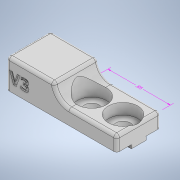
# Autodesk Inventor part: Mount Female V3
Saved by Autodesk Inventor 2020 (Build 240168000, 168)
## iProperties
Created: 2020-01-27
Part Number: Mount Female V3
Material: Generic
Document SubType Name: Modeling
Designer: maple
Density: 1 g/cm^3
Appearance: Default
Author: maple
Autodesk Inventor part; units mm, degrees
ref_plane "YZ Plane" through (0, 0, 0) normal (1, 0, 0) x (0, 1, 0)
ref_plane "XZ Plane" through (0, 0, 0) normal (0, 1, 0) x (-1, 0, 0)
ref_plane "XY Plane" through (0, 0, 0) normal (0, 0, 1) x (1, 0, 0)
sketch "Sketch1" plane through (0, 0, 0) normal (0, 1, 0) x (-1, 0, 0)
  line L0 (0, 0) -> (-38.1, 0)
  line L1 (-38.1, 0) -> (-38.1, -15.24)
  line L2 (-38.1, -15.24) -> (0, -15.24)
  line L3 (0, -15.24) -> (0, 0)
  dimension "d0" = 38.1
  dimension "d1" = 15.24
  constraints: 8 end point, 2 parallel, 1 horizontal, 1 perpendicular
  measures "d0" distance of L2.end L1.end
  measures "d1" distance of L1.end L0.end
extrude "Extrusion1" add sketch "Sketch1" along normal blind 5.08
sketch "Sketch2" plane through (0, 5.08, 0) normal (0, 1, 0) x (1, 0, 0)
  line L0 (0, 0) -> (16.51, 0)
  line L1 (16.51, 0) -> (16.51, 15.24)
  line L2 (16.51, 15.24) -> (0, 15.24)
  line L3 (0, 15.24) -> (0, 0)
  dimension "d4" = 16.51
  dimension "d5" = 15.24
  constraints: 8 end point, 2 parallel, 1 horizontal, 1 perpendicular
  measures "d4" distance of L2.end L1.end
  measures "d5" distance of L1.end L0.end
extrude "Extrusion2" add sketch "Sketch2" along normal blind 5.08
sketch "Sketch3" plane through (0, 0, -15.24) normal (-1, 0, 0) x (0, 0, 1)
  line L0 (0, 10.16) -> (15.24, 10.16) projected
  line L1 (7.62, 10.16) -> (7.62, 8.89)
  line L2 (7.62, 8.89) -> (2.54, 8.89)
  line L3 (2.54, 8.89) -> (2.54, 3.81)
  line L4 (2.54, 3.81) -> (12.7, 3.81)
  line L5 (12.7, 3.81) -> (12.7, 8.89)
  line L6 (12.7, 8.89) -> (7.62, 8.89)
  point P0 (15.24, 0)
  dimension "d8" = 1.27
  dimension "d9" = 5.08
  dimension "d10" = 5.08
  dimension "d11" = 10.16
  dimension "d12" = 90
  dimension "d13" = 5.08
  constraints: 12 end point, 2 perpendicular, 1 horizontal, 1 midpoint, 1 point on line, 1 vertical
  measures "d8" distance of L1.start L1.end
  measures "d9" distance of L1.end L2.end
  measures "d10" distance of L2.end L3.end
  measures "d11" distance of L3.end L4.end
  measures "d12" angle of L4 L3
  measures "d13" distance of L4.end L5.end
extrude "Extrusion3" cut sketch "Sketch3" against normal blind 15.24
sketch "Sketch4" plane through (0, 5.08, 0) normal (0, 1, 0) x (1, 0, 0)
  line L0 (38.1, 0) -> (38.1, 15.24) projected
  line L1 (38.1, 7.62) -> (32.7025, 7.62)
  line L2 (32.7025, 7.62) -> (27.305, 7.62)
  line L3 (27.305, 7.62) -> (21.8948, 7.62)
  point P0 (0, 0)
  dimension "d19" = 5.3975
  dimension "d20" = 5.3975
  dimension "d21" = 180
  dimension "d22" = 5.4102
  dimension "d23" = 180
  constraints: 6 end point, 2 collinear, 1 horizontal, 1 midpoint
  measures "d19" distance of L1.start L1.end
  measures "d20" distance of L1.end L2.end
  measures "d21" angle of L2 L1
  measures "d22" distance of L2.end L3.end
  measures "d23" angle of L3 L2
sketch "Sketch5" plane through (0, 0, 0) normal (0, -1, 0) x (1, 0, 0)
  line L0 (0, -15.24) -> (0, 0) projected
  line L1 (0, -7.62) -> (0, -10.16)
  line L2 (0, -10.16) -> (0, -5.08)
  line L3 (0, -5.08) -> (38.1, -5.08)
  line L4 (38.1, -5.08) -> (38.1, -10.16)
  line L5 (38.1, -10.16) -> (0, -10.16)
  line L6 (0, -10.16) -> (0, -5.08)
  dimension "d31" = 2.54
  dimension "d32" = 5.08
  dimension "d33" = 38.1
  dimension "d34" = 5.08
  constraints: 12 end point, 2 parallel, 2 point on line, 1 horizontal, 1 midpoint, 1 perpendicular
  measures "d31" distance of L1.start L1.end
  measures "d32" distance of L1.end L2.end
  measures "d33" distance of L4.end L5.end
  measures "d34" distance of L3.end L4.end
extrude "Extrusion4" add sketch "Sketch5" along normal blind 1.27
hole "Hole2" at (32.7025, 5.08, -7.62) at (21.8948, 5.08, -7.62) direction (0, -1, 0) diameter 5.08 end through all counterbore diameter 10.16 counterbore depth 3.81
fillet "Fillet1" radius 5.08 1 edges at (16.51, 5.08, -7.62)
fillet "Fillet2" radius 1.016 13 edges at (8.255, 10.16, 0) (8.255, 10.16, -15.24) (0, 5.08, -15.24) (0, 10.16, -7.62) (0, 5.08, 0) (16.51, 10.16, -7.62) (17.9979, 6.5679, 0) (29.845, 5.08, 0) (17.9979, 6.5679, -15.24) (29.845, 5.08, -15.24) (38.1, 5.08, -7.62) (38.1, 2.54, 0) (38.1, 2.54, -15.24)
fillet "Fillet3" radius 0.508 4 edges at (0, 3.81, -7.62) (0, 6.35, -2.54) (0, 6.35, -12.7) (0, 8.89, -7.62)
sketch "Sketch6" plane through (1.016, 0, 0) normal (0, 0, 1) x (1, 0, 0)
  line L0 (0.1598, 7.1739) -> (9.3236, 7.1739) construction
  line L1 (9.3236, 7.1739) -> (9.3236, 1.8798) construction
  line L2 (9.3236, 1.8798) -> (0.1598, 1.8798) construction
  line L3 (0.1598, 1.8798) -> (0.1598, 7.1739) construction
  line L4 (3.7352, 6.4319) -> (2.4261, 2.6219)
  line L5 (2.4261, 2.6219) -> (1.4288, 2.6219)
  line L6 (1.4288, 2.6219) -> (0.1197, 6.4319)
  line L7 (0.1197, 6.4319) -> (1.1108, 6.4319)
  line L8 (1.1108, 6.4319) -> (1.9413, 3.8476)
  line L9 (1.9413, 3.8476) -> (2.7688, 6.4319)
  line L10 (2.7688, 6.4319) -> (3.7352, 6.4319)
  spline S0 degree 2 poles (6.7856, 3.7766) (6.7856, 3.4956) (6.5788, 3.0356) (6.3781, 2.8751) knots 0 0 0 1 2 2 2
  spline S1 degree 2 poles (6.3781, 2.8751) (6.1774, 2.7145) (5.6309, 2.5416) (5.2388, 2.5416) knots 0 0 0 1 2 2 2
  spline S2 degree 2 poles (5.2388, 2.5416) (4.7942, 2.5416) (4.1582, 2.6898) (3.9575, 2.7824) knots 0 0 0 1 2 2 2
  line L11 (3.9575, 2.7824) -> (3.9575, 3.6099)
  line L12 (3.9575, 3.6099) -> (4.0501, 3.6099)
  spline S3 degree 2 poles (4.0501, 3.6099) (4.26, 3.4771) (4.8251, 3.2795) (5.0597, 3.2795) knots 0 0 0 1 2 2 2
  spline S4 degree 2 poles (5.0597, 3.2795) (5.1986, 3.2795) (5.5228, 3.3289) (5.634, 3.4092) knots 0 0 0 1 2 2 2
  spline S5 degree 2 poles (5.634, 3.4092) (5.7204, 3.474) (5.8254, 3.6624) (5.8254, 3.8322) knots 0 0 0 1 2 2 2
  spline S6 degree 2 poles (5.8254, 3.8322) (5.8254, 4.002) (5.6772, 4.1842) (5.5537, 4.2274) knots 0 0 0 1 2 2 2
  spline S7 degree 2 poles (5.5537, 4.2274) (5.4302, 4.2706) (5.0875, 4.2799) (4.9547, 4.2799) knots 0 0 0 1 2 2 2
  line L13 (4.9547, 4.2799) -> (4.7911, 4.2799)
  line L14 (4.7911, 4.2799) -> (4.7911, 4.9499)
  line L15 (4.7911, 4.9499) -> (4.9424, 4.9499)
  spline S8 degree 2 poles (4.9424, 4.9499) (5.1153, 4.9499) (5.4086, 4.9807) (5.5105, 5.0271) knots 0 0 0 1 2 2 2
  spline S9 degree 2 poles (5.5105, 5.0271) (5.6124, 5.0765) (5.7266, 5.2494) (5.7266, 5.3976) knots 0 0 0 1 2 2 2
  spline S10 degree 2 poles (5.7266, 5.3976) (5.7266, 5.5149) (5.6185, 5.66) (5.5414, 5.7001) knots 0 0 0 1 2 2 2
  spline S11 degree 2 poles (5.5414, 5.7001) (5.4487, 5.7464) (5.2017, 5.7773) (5.1153, 5.7773) knots 0 0 0 1 2 2 2
  spline S12 degree 2 poles (5.1153, 5.7773) (4.9763, 5.7773) (4.683, 5.7125) (4.5472, 5.66) knots 0 0 0 1 2 2 2
  spline S13 degree 2 poles (4.5472, 5.66) (4.4391, 5.6199) (4.2045, 5.4902) (4.1489, 5.4562) knots 0 0 0 1 2 2 2
  line L16 (4.1489, 5.4562) -> (4.0686, 5.4562)
  line L17 (4.0686, 5.4562) -> (4.0686, 6.2713)
  spline S14 degree 2 poles (4.0686, 6.2713) (4.2662, 6.3547) (4.9331, 6.5122) (5.282, 6.5122) knots 0 0 0 1 2 2 2
  spline S15 degree 2 poles (5.282, 6.5122) (5.6216, 6.5122) (6.1218, 6.3948) (6.2978, 6.2806) knots 0 0 0 1 2 2 2
  spline S16 degree 2 poles (6.2978, 6.2806) (6.4923, 6.1602) (6.6868, 5.7897) (6.6868, 5.5581) knots 0 0 0 1 2 2 2
  spline S17 degree 2 poles (6.6868, 5.5581) (6.6868, 5.2308) (6.3102, 4.743) (6.0014, 4.672) knots 0 0 0 1 2 2 2
  line L18 (6.0014, 4.672) -> (6.0014, 4.6349)
  spline S18 degree 2 poles (6.0014, 4.6349) (6.1373, 4.6164) (6.3966, 4.5176) (6.5201, 4.4065) knots 0 0 0 1 2 2 2
  spline S19 degree 2 poles (6.5201, 4.4065) (6.6343, 4.3077) (6.7856, 3.9927) (6.7856, 3.7766) knots 0 0 0 1 2 2 2
  point P0 (-1.016, 0)
  constraints: 2 other
emboss "Emboss1" sketch "Sketch6" operation cut depth 0.508 direction (0, 0, -1)
body "Solid1"
